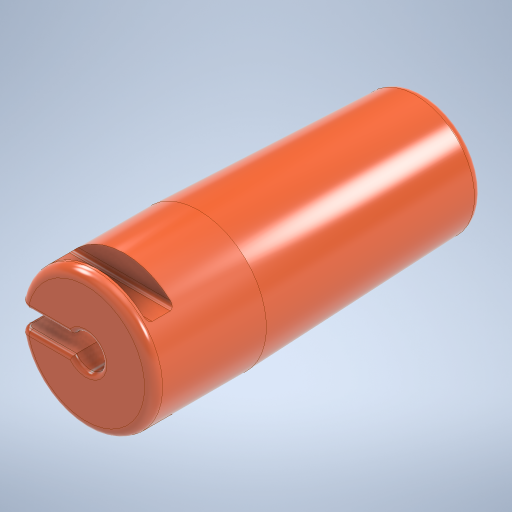
# Autodesk Inventor part: Ferula hembra Fiber Op
Saved by Autodesk Inventor 2024.2 (Build 282272000, 272)
## iProperties
Created: 2025-06-04
Part Number: Ferula hembra Fiber Op
Material: Phenolic Resin
Document SubType Name: Modeling
Designer: ja.restrepo1
Density: 1.38 g/cm^3
Appearance: Smooth - Light Orange
Author: ja.restrepo1
Autodesk Inventor part; units mm, degrees
ref_plane "YZ Plane" through (0, 0, 0) normal (1, 0, 0) x (0, 1, 0)
ref_plane "XZ Plane" through (0, 0, 0) normal (0, 1, 0) x (-1, 0, 0)
ref_plane "XY Plane" through (0, 0, 0) normal (0, 0, 1) x (1, 0, 0)
sketch "Sketch1" plane through (0, 0, 0) normal (1, 0, 0) x (0, 1, 0)
  line L0 (0.725, 5) -> (0.725, 7.5)
  line L1 (0.725, 7.5) -> (3, 7.5)
  line L2 (3, 7.5) -> (3, -7.5)
  line L3 (3, -7.5) -> (2, -7.5)
  line L4 (2, 5) -> (0.725, 5)
  line L5 (0, 10.8962) -> (0, -10.8962) construction
  line L6 (2, -7.5) -> (2, 5)
  point P0 (0, 0)
  point P1 (0, 0)
  point P2 (3, 0)
  dimension "d0" = 15
  dimension "d2" = 0.725
  dimension "d3" = 2.5
  dimension "d4" = 3
  dimension "d14" = 2
  constraints: 14 end point, 3 perpendicular, 2 coincident, 2 midpoint, 2 vertical, 1 horizontal, 1 horizontal alignment, 1 parallel
  measures "d0" distance of L1.end L2.end
  measures "d2" distance between parallel lines of L0 L5
  measures "d3" distance of L0.start L0.end
  measures "d4" distance between parallel lines of L2 L5
  measures "d14" horizontal distance of point (0, 0) L4.start
revolve "Revolution1" add sketch "Sketch1" angle 360 about axis through (0, 0, 10.8962) along (0, 0, -1)
chamfer "Chamfer1" distance 0.2 angle 45 1 edges at (0, -0.725, 5)
chamfer "Chamfer2" distance 0.4 distance2 10 1 edges at (0, -3, -7.5) measured on face at (0, -2.5, -7.5)
fillet "Fillet1" radius 0.4 4 edges at (0, -3, 7.5) (0, -2.6, -7.5) (0, -2, -7.5) (0, -2, 5)
sketch "Sketch2" plane through (0, 0, 0) normal (1, 0, 0) x (0, 1, 0)
  line L0 (0.4, 7.5) -> (-0.4, 7.5)
  line L1 (-0.4, 7.5) -> (-0.4, -7.5)
  line L2 (-0.4, -7.5) -> (0.4, -7.5)
  line L3 (0.4, -7.5) -> (0.4, 7.5)
  line L4 (-2.6, 7.5) -> (2.6, 7.5) projected
  point P0 (0, 0)
  point P1 (0, -7.5)
  dimension "d15" = 0.8
  dimension "d16" = 15
  constraints: 8 end point, 2 parallel, 1 collinear, 1 horizontal, 1 midpoint, 1 perpendicular, 1 vertical alignment
  measures "d15" distance of L2.end L1.end
  measures "d16" distance of L1.end L0.end
extrude "Extrusion1" cut sketch "Sketch2" against normal blind 10
pattern_circular "Circular Pattern1" [suppressed]
fillet "Fillet2" radius 0.2 9 edges at (0.725, 0, 7.5) (-2.8548, -0.4, 7.383) (-2.9732, -0.4, 4.8) (-1.5869, -0.4, 7.5) (-2.8548, 0.4, 7.383) (-2.9732, 0.4, 4.8) (-1.5869, 0.4, 7.5) (-2.7722, -0.4, -2.4763) (-2.7722, 0.4, -2.4763)
sketch "Sketch3" plane through (0, 0, 0) normal (1, 0, 0) x (0, 1, 0)
  line L0 (-3.5, 7) -> (-2, 7)
  line L1 (-2, 7) -> (-2, 5.8)
  line L2 (-2, 5.8) -> (-3.5, 5.8)
  line L3 (-3.5, 5.8) -> (-3.5, 7)
  line L4 (2, 7) -> (3.5, 7)
  line L5 (3.5, 7) -> (3.5, 5.8)
  line L6 (3.5, 5.8) -> (2, 5.8)
  line L7 (2, 5.8) -> (2, 7)
  line L8 (-2.6, 7.5) -> (2.6, 7.5) projected
  line L9 (-2, 6.4) -> (2, 6.4) construction
  point P0 (0, 0)
  point P1 (0.6, 7.5)
  point P2 (-0.6, 7.5)
  point P3 (0, 6.4)
  dimension "d25" = 1.5
  dimension "d26" = 1.2
  dimension "d27" = 1.5
  dimension "d28" = 0.5
  dimension "d29" = 4
  constraints: 18 end point, 4 parallel, 3 midpoint, 2 horizontal, 2 perpendicular, 2 point on line, 1 vertical alignment
  measures "d25" distance of L1.end L2.end
  measures "d26" distance of L0.end L1.end
  measures "d27" distance of L5.end L6.end
  measures "d28" distance between parallel lines of L0 L8
  measures "d29" distance of L9.start L9.end
extrude "cajas extractoras" cut sketch "Sketch3" along normal through all both and the other way through all
fillet "Fillet3" radius 0.2 4 edges at (0, -2, 5.8) (0, 2, 5.8) (0, -2, 7) (0, 2, 7)
body "Solid1"
